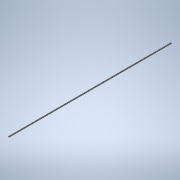
# Autodesk Inventor part: carbon_spar
Saved by Autodesk Inventor 2021 (Build 250183000, 183)
## iProperties
Created: 2020-12-08
Part Number: carbon_spar
Material: CFRP
Document SubType Name: Modeling
Designer: victo
Mass: 1.19434 g
Surface Area: 33.6348 cm^2
Volume: 0.8352 cm^3
Density: 1.43 g/cm^3
Appearance: Carbon Fiber
Author: victo
Autodesk Inventor part; units mm, degrees
ref_plane "YZ Plane" through (0, 0, 0) normal (1, 0, 0) x (0, 1, 0)
ref_plane "XZ Plane" through (0, 0, 0) normal (0, 1, 0) x (-1, 0, 0)
sketch "Sketch1" plane through (0, 0, 0) normal (0, 0, 1) x (1, 0, 0)
  line L0 (0, 0) -> (2.9, 0)
  line L1 (2.9, 0) -> (2.9, 0.6)
  line L2 (2.9, 0.6) -> (0, 0.6)
  line L3 (0, 0.6) -> (0, 0)
  dimension "d0" = 0.6
  dimension "d1" = 2.9
  constraints: 8 end point, 2 parallel, 1 horizontal, 1 perpendicular
  measures "d0" distance of L0.end L1.end
  measures "d1" distance of L1.end L2.end
extrude "Extrusion1" add sketch "Sketch1" along normal blind 480
ref_plane "Work Plane1" through (0, 0, 240) normal (0, 0, 1) x (1, 0, 0)
body "Solid1"
